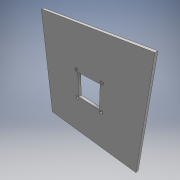
# Autodesk Inventor part: Bassic Vehicle Chassis
Saved by Autodesk Inventor 2016 (Build 200138000, 138)
## iProperties
Created: 2016-02-20
Part Number: Bassic Vehicle Chassis
Material: Generic
Document SubType Name: Modeling
Designer: Kenneth Daniel
Density: 1 g/cm^3
Appearance: Default
Author: Kenneth Daniel
Autodesk Inventor part; units mm, degrees
ref_plane "YZ Plane" through (0, 0, 0) normal (1, 0, 0) x (0, 1, 0)
ref_plane "XZ Plane" through (0, 0, 0) normal (0, 1, 0) x (-1, 0, 0)
ref_plane "XY Plane" through (0, 0, 0) normal (0, 0, 1) x (1, 0, 0)
sketch "Sketch1" plane through (0, 0, 0) normal (0, 1, 0) x (-1, 0, 0)
  line L0 (-175, 175) -> (-175, -175)
  line L1 (-175, -175) -> (175, -175)
  line L2 (175, -175) -> (175, 175)
  line L3 (175, 175) -> (-175, 175)
  line L4 (-175, 175) -> (175, -175) construction
  line L5 (-175, -175) -> (175, 175) construction
  point P0 (0, 0)
  dimension "d0" = 350
  dimension "d1" = 350
  constraints: 12 end point, 2 midpoint, 2 parallel, 1 perpendicular, 1 vertical
  measures "d0" distance of L1.end L2.end
  measures "d1" distance of L0.end L1.end
extrude "Extrusion1" add sketch "Sketch1" along normal blind 10
sketch "Sketch2" plane through (0, 10, 0) normal (0, 1, 0) x (1, 0, 0)
  line L0 (175, -175) -> (175, 175) projected
  line L1 (175, 175) -> (-175, 175) projected
  line L2 (-175, 175) -> (-175, -175) projected
  line L3 (-175, -175) -> (175, -175) projected
  line L4 (-175, 175) -> (175, -175) construction
  line L5 (-175, -175) -> (175, -175) construction
  line L6 (-175, -175) -> (161.7326, 161.7326) construction
  line L7 (40, -40) -> (40, 40)
  line L8 (40, 40) -> (-40, 40)
  line L9 (-40, 40) -> (-40, -40)
  line L10 (-40, -40) -> (40, -40)
  line L11 (40, -40) -> (-40, 40) construction
  line L12 (40, 40) -> (-40, -40) construction
  point P0 (0, 0)
  dimension "d4" = 80
  dimension "d5" = 80
  constraints: 16 end point, 2 midpoint, 2 parallel, 2 perpendicular, 1 vertical
  measures "d4" distance of L8.end L9.end
  measures "d5" distance of L7.end L8.end
extrude "Extrusion2" cut sketch "Sketch2" against normal blind 10 contours L10 L9 L8 L7
sketch "Sketch3" plane through (0, 10, 0) normal (0, 1, 0) x (1, 0, 0)
  line L0 (40, -40) -> (-40, -40) projected
  point P0 (0, 0)
sketch "Sketch4" plane through (0, 10, 0) normal (0, 1, 0) x (1, 0, 0)
  line L0 (40, -40) -> (-40, -40) construction
  line L1 (45, -40) -> (50, -40) construction
  line L2 (45, -40) -> (50, -40)
  line L3 (50, -40) -> (50, -50)
  line L4 (50, -50) -> (40, -50)
  line L5 (40, 40) -> (40, -40) projected
  line L6 (40, -50) -> (40, -45)
  line L7 (45, -45) -> (40, -45)
  line L8 (45, -45) -> (45, -40)
  line L9 (111.0748, 0) -> (-96.7509, 0) construction
  line L10 (0, -82.157) -> (0, 67.3265) construction
  line L11 (45, 40) -> (50, 40)
  line L12 (50, 40) -> (50, 50)
  line L13 (50, 50) -> (40, 50)
  line L14 (40, 50) -> (40, 45)
  line L15 (45, 45) -> (40, 45)
  line L16 (45, 45) -> (45, 40)
  line L17 (-45, -40) -> (-50, -40)
  line L18 (-50, -40) -> (-50, -50)
  line L19 (-50, -50) -> (-40, -50)
  line L20 (-40, -50) -> (-40, -45)
  line L21 (-45, -45) -> (-40, -45)
  line L22 (-45, -45) -> (-45, -40)
  line L23 (-50, 40) -> (-50, 50)
  line L24 (-45, 45) -> (-45, 40)
  line L25 (-45, 45) -> (-40, 45)
  line L26 (-40, 50) -> (-40, 45)
  line L27 (-50, 50) -> (-40, 50)
  line L28 (-45, 40) -> (-50, 40)
  point P0 (0, 0)
  dimension "d10" = 10
  dimension "d11" = 10
  dimension "d12" = 10
  dimension "d14" = 5
  dimension "d15" = 5
  constraints: 54 end point, 18 symmetric about line, 3 horizontal, 1 collinear, 1 perpendicular, 1 point on line, 1 vertical
  measures "d10" distance of L0.start L2.end
  measures "d11" distance of L2.end L3.end
  measures "d12" distance of L3.end L4.end
  measures "d14" distance of L6.end L7.start
  measures "d15" distance of L1.start L7.start
extrude "Extrusion3" cut sketch "Sketch4" against normal blind 10
sketch "Sketch5" plane through (0, 10, 0) normal (0, 1, 0) x (1, 0, 0)
  line L0 (-45, -45) -> (-40, -45) projected
  line L1 (40, -45) -> (-40, -45)
  line L2 (-40, -45) -> (-40, -50) projected
  line L3 (-40, -45) -> (-40, -50)
  line L4 (40, -50) -> (40, -45) projected
  line L5 (-40, -50) -> (40, -50)
  point P0 (0, 0)
  constraints: 6 end point, 2 perpendicular, 1 horizontal
extrude "Extrusion4" cut sketch "Sketch5" against normal blind 5
mirror "Mirror1" about plane through (0, 0, 0) normal (0, 0, 1) of "Extrusion4"
body "Solid1"
